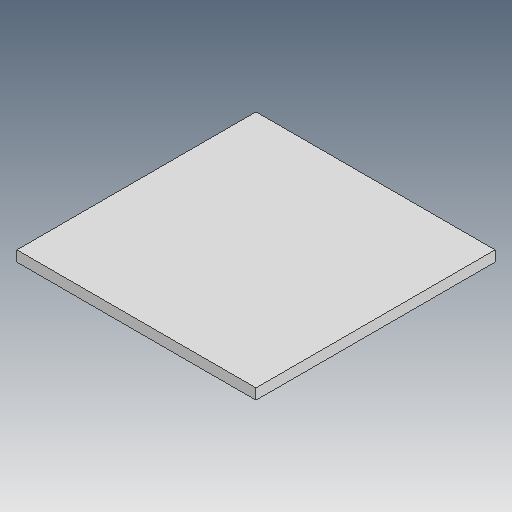
# Autodesk Inventor part: base_plate
Saved by Autodesk Inventor 2025.1 (Build 291241000, 241)
## iProperties
Created: 2026-06-20
Part Number: base_plate
Material: Generic
Document SubType Name: Modeling
Designer: Aiden
Density: 1 g/cm^3
Appearance: Default
Author: Aiden
Autodesk Inventor part; units mm, degrees
ref_plane "YZ Plane" through (0, 0, 0) normal (1, 0, 0) x (0, 1, 0)
ref_plane "XZ Plane" through (0, 0, 0) normal (0, 1, 0) x (-1, 0, 0)
ref_plane "XY Plane" through (0, 0, 0) normal (0, 0, 1) x (1, 0, 0)
sketch "Sketch1" plane through (0, 0, 0) normal (0, 1, 0) x (-1, 0, 0)
  line L0 (112.5, 112.5) -> (-112.5, 112.5)
  line L1 (-112.5, 112.5) -> (-112.5, -112.5)
  line L2 (-112.5, -112.5) -> (112.5, -112.5)
  line L3 (112.5, -112.5) -> (112.5, 112.5)
  line L4 (112.5, 112.5) -> (-112.5, -112.5) construction
  line L5 (-112.5, 112.5) -> (112.5, -112.5) construction
  point P0 (0, 0)
  dimension "d0" = 225
  dimension "d1" = 225
  constraints: 12 end point, 2 midpoint, 2 parallel, 1 horizontal, 1 perpendicular
  measures "d0" distance of L2.end L0.start
  measures "d1" distance of L1.end L2.end
extrude "Extrusion1" add sketch "Sketch1" along normal blind 10
body "Solid1"
